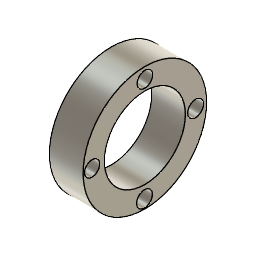
3rd project (Autodesk Fusion 360 design; units mm, degrees)
part number: 2025-07-20-15-59-38-084
Autodesk Fusion 360 part; units mm, degrees
sketch "Sketch1" plane through (0, 0, 0) normal (1, 0, 0) x (0, 1, 0)
  circle A0 centre (0, 0) radius 1.4616
  circle A1 centre (0, 0) radius 0.9577
  circle A2 centre (0, 1.2) radius 0.1839
  circle A3 centre (1.2, 0) radius 0.1879
  circle A4 centre (-1.2505, -0.0025) radius 0.1794
  circle A5 centre (-0.0098, -1.2481) radius 0.1875
  constraint coincident A0.centre A1.centre
  constraint concentric A0 A1
extrude "Extrude1" add sketch "Sketch1" along normal blind 0.8
